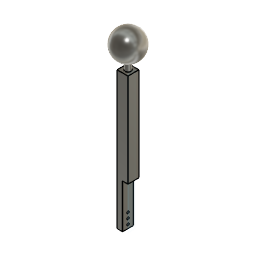
BRAS1 (Autodesk Fusion 360 design; units mm, degrees)
Autodesk Fusion 360 part; units mm, degrees
sketch "Esquisse1" plane through (0, 0, 0) normal (1, 0, 0) x (0, 1, 0)
sphere "SpherePrimitive1" add diameter 40 placed x (0, 1, 0) y (0, 0, 1) z (1, 0, 0) at (0, 0, 0)
sketch "Esquisse2" plane through (0, 0, 0) normal (0, 0, 1) x (1, 0, 0)
  circle A0 centre (0, 0) radius 2.5
  dimension "d2" = 5
  constraint coincident A0.centre origin
  measures "d2" diameter of A0
extrude "Extrusion1" add sketch "Esquisse2" against normal blind 30
box "BoitePrimitive1" cut length 10 width 10 height 1 placed x (0, 1, 0) y (-1, 0, 0) z (0, 0, 1) at (5, -5, 0)
sketch "Esquisse4" plane through (0, 0, 0) normal (0, 0, 1) x (1, 0, 0)
box "BoitePrimitive2" add length 10 width 10 height 188.75 placed x (0, 1, 0) y (1, 0, 0) z (0, 0, -1) at (-5, -5, -30)
sketch "Esquisse6" plane through (0, 0, -218.75) normal (0, 0, -1) x (1, 0, 0)
  line L0 (-5, -5) -> (5, -5)
  line L1 (5, -5) -> (5, 5)
  line L2 (5, 5) -> (-5, 5)
  line L3 (-5, 5) -> (-5, -5)
extrude "Extrusion2" add sketch "Esquisse6" against normal blind 17.5
move_face "DécalerLesFaces1" offset -1.307 1 faces at (1.6667, -1.6667, -218.75)
sketch "Esquisse7" plane through (5, 0, 0) normal (1, 0, 0) x (0, 1, 0)
  line L0 (5, -217.443) -> (5, -30)
  line L1 (5, -30) -> (-5, -30)
  line L2 (-5, -30) -> (-5, -217.443)
  line L3 (-5, -217.443) -> (5, -217.443)
hole "Perçage1" at (5, 0.0021, -198.2029) direction (-1, 0, 0) diameter 3 depth 10 tip angle 118
hole "Perçage2" at (5, -0.0059, -205.3239) direction (-1, 0, 0) diameter 3 depth 10 tip angle 118
hole "Perçage3" at (5, 0.0869, -212.4423) direction (-1, 0, 0) diameter 3 depth 10 tip angle 118
sketch "Esquisse8" plane through (0, -5, 0) normal (0, -1, 0) x (1, 0, 0)
  line L0 (5, -217.443) -> (5, -30)
  line L1 (5, -30) -> (-5, -30)
  line L2 (-5, -30) -> (-5, -217.443)
  line L3 (-5, -217.443) -> (5, -217.443)
  line L4 (5, -217.443) -> (0, -217.443)
  line L5 (0, -217.443) -> (0, -157.443)
  line L6 (0, -157.443) -> (5, -157.443)
  line L7 (5, -157.443) -> (5, -217.443)
  dimension "d30" = 60
  constraint horizontal L4
  constraint vertical L5
  constraint horizontal L6
  constraint vertical L7
  constraint coincident L0.start L3.end
  measures "d30" distance of L0.start L6.end
extrude "Extrusion3" cut sketch "Esquisse8" against normal blind 10 contours L0 L3 L4 L5 L6 L7
move_face "DécalerLesFaces2" offset 1.5 1 faces at (2.4876, -0.2489, -23.2288)
move_face "DécalerLesFaces3" offset 5 1 faces at (0, -5, -72.481)
move_face "DécalerLesFaces4" offset 5 1 faces at (0, 5, -72.481)
move_face "DécalerLesFaces5" offset 5 1 faces at (-5, -0.062, -85.5716)
move_face "DécalerLesFaces6" offset 5 1 faces at (5, 3.3333, -114.962)
move_face "DécalerLesFaces7" offset -2.5 1 faces at (10, 3.3333, -114.962)
move_face "DécalerLesFaces8" offset -2.5 1 faces at (-0.8333, -10, -72.481)
move_face "DécalerLesFaces9" offset -2.5 1 faces at (-0.8333, 10, -72.481)
move_face "DécalerLesFaces10" offset -2.5 1 faces at (-10, 0.0007, -85.5676)
equation "d12 = 200 mm - 30 mm + 18.75 mm"
equation "d15 = -202.374 mm - 20 mm - 12.626 mm + 17.5 mm + 200 mm"
